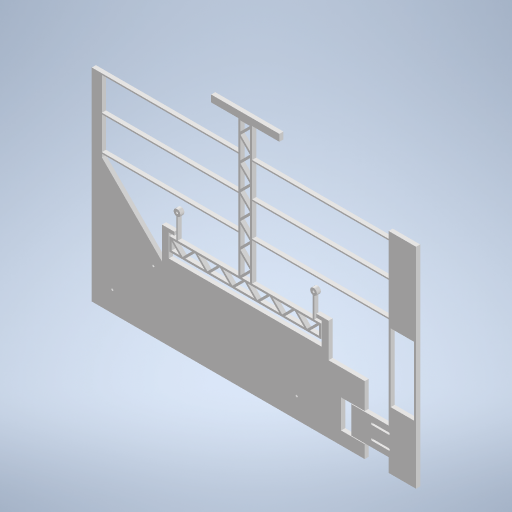
# Autodesk Inventor part: Inverter
Saved by Autodesk Inventor 2023 (Build 270158000, 158)
## iProperties
Created: 2023-05-11
Part Number: Inverter
Material: Generic
Document SubType Name: Modeling
Designer: Nathann
Density: 1 g/cm^3
Appearance: Default
Author: Nathann
Autodesk Inventor part; units mm, degrees
ref_plane "YZ Plane" through (0, 0, 0) normal (1, 0, 0) x (0, 1, 0)
ref_plane "XZ Plane" through (0, 0, 0) normal (0, 1, 0) x (-1, 0, 0)
ref_plane "XY Plane" through (0, 0, 0) normal (0, 0, 1) x (1, 0, 0)
sketch "Sketch1" plane through (0, 0, 0) normal (0, 0, 1) x (1, 0, 0)
  line L0 (0, 0) -> (-420, 0)
  line L1 (-420, 0) -> (-420, 350)
  line L2 (-420, 350) -> (0, 350)
  line L3 (0, 350) -> (0, 98.9027)
  line L4 (-98.9528, 98.9027) -> (-175.0251, 174.9749)
  line L5 (-175.0251, 174.9749) -> (0, 350)
  line L6 (-75.0251, 174.899) -> (-275.025, 174.899)
  circle A0 centre (-275.025, 174.899) radius 1.5
  circle A1 centre (-275.025, 174.899) radius 5
  circle A2 centre (-75.0251, 174.899) radius 5
  circle A3 centre (-75.0251, 174.899) radius 1.5
  line L7 (-274.025, 170) -> (-276.025, 170)
  line L8 (-276.025, 170) -> (-276.025, 140)
  line L9 (-276.025, 140) -> (-274.025, 140)
  line L10 (-274.025, 140) -> (-274.025, 170)
  line L11 (-74.0251, 170) -> (-76.0251, 170)
  line L12 (-76.0251, 170) -> (-76.0251, 140)
  line L13 (-76.0251, 140) -> (-74.0251, 140)
  line L14 (-74.0251, 140) -> (-74.0251, 170)
  line L15 (-64.0251, 140) -> (-286.025, 140)
  line L16 (-286.025, 140) -> (-286.025, 120)
  line L17 (-286.025, 120) -> (-64.0251, 120)
  line L18 (-64.0251, 120) -> (-64.0251, 140)
  line L19 (-165.0251, 140) -> (-185.0251, 140)
  line L20 (-185.0251, 140) -> (-185.0251, 340)
  line L21 (-185.0251, 340) -> (-165.0251, 340)
  line L22 (-165.0251, 340) -> (-165.0251, 140)
  line L23 (-185, 339) -> (-185.0251, 340)
  line L24 (-185.0251, 194.899) -> (-385.0251, 194.899)
  line L25 (-385.0251, 194.899) -> (-385.0251, 196.899)
  line L26 (-385.0251, 196.899) -> (-185.0251, 196.899)
  line L27 (-185.0251, 196.899) -> (-185.0251, 194.899)
  line L28 (-185.0251, 296.899) -> (-385.0251, 296.899)
  line L29 (-385.0251, 296.899) -> (-385.0251, 294.899)
  line L30 (-385.0251, 294.899) -> (-185.0251, 294.899)
  line L31 (-185.0251, 294.899) -> (-185.0251, 296.899)
  line L32 (-225.0251, 350) -> (-125.0251, 350)
  line L33 (-125.0251, 350) -> (-125.0251, 340)
  line L34 (-125.0251, 340) -> (-225.0251, 340)
  line L35 (-225.0251, 340) -> (-225.0251, 350)
  line L36 (-165.0251, 294.899) -> (34.9749, 294.899)
  line L37 (34.9749, 294.899) -> (34.9749, 296.899)
  line L38 (34.9749, 296.899) -> (-165.0251, 296.899)
  line L39 (-165.0251, 296.899) -> (-165.0251, 294.899)
  line L40 (0, 0) -> (135.1933, 0)
  line L41 (135.1933, 0) -> (135.1933, 350)
  line L42 (135.1933, 350) -> (0, 350)
  line L43 (0, 350) -> (0, 98.9027)
  line L44 (-165.0251, 196.899) -> (34.9749, 196.899)
  line L45 (34.9749, 196.899) -> (34.9749, 194.899)
  line L46 (34.9749, 194.899) -> (-165.0251, 194.899)
  line L47 (-165.0251, 194.899) -> (-165.0251, 196.899)
  line L48 (-420, 350) -> (-385, 350)
  line L49 (-385, 350) -> (-385, 98.9027)
  line L50 (-385, 98.9027) -> (-420, 98.9027)
  line L51 (-420, 98.9027) -> (-420, 350)
  line L52 (135.1933, 98.9027) -> (135.1933, 0)
  line L53 (135.1933, 0) -> (-420, 0)
  line L54 (-420, 0) -> (-420, 98.9027)
  line L55 (-185.0251, 246.899) -> (-385, 246.899)
  line L56 (-385, 246.899) -> (-385, 244.899)
  line L57 (-385, 244.899) -> (-185.0251, 244.899)
  line L58 (-185.0251, 244.899) -> (-185.0251, 246.899)
  line L59 (-165.0251, 246.899) -> (35, 246.899)
  line L60 (35, 246.899) -> (35, 244.899)
  line L61 (35, 244.899) -> (-165.0251, 244.899)
  line L62 (-165.0251, 244.899) -> (-165.0251, 246.899)
  line L63 (35, 306.899) -> (75, 306.899)
  line L64 (75, 306.899) -> (75, 184.899)
  line L65 (75, 184.899) -> (35, 184.899)
  line L66 (35, 184.899) -> (35, 306.899)
  line L67 (35, 184.899) -> (38, 184.899)
  line L68 (38, 184.899) -> (38, 84.899)
  line L69 (38, 84.899) -> (35, 84.899)
  line L70 (35, 84.899) -> (35, 184.899)
  line L71 (75, 184.899) -> (72, 184.899)
  line L72 (72, 184.899) -> (72, 84.899)
  line L73 (72, 84.899) -> (75, 84.899)
  line L74 (75, 84.899) -> (75, 184.899)
  line L75 (75, 84.899) -> (35, 84.899)
  line L76 (35, 84.899) -> (35, 0)
  line L77 (35, 0) -> (75, 0)
  line L78 (75, 0) -> (75, 84.899)
  line L79 (-420, 98.9027) -> (0, 98.9027)
  line L80 (35, 60) -> (-19.6162, 60)
  line L81 (-19.6162, 60) -> (-19.6162, 20)
  line L82 (-19.6162, 20) -> (35, 20)
  line L83 (35, 20) -> (35, 60)
  line L84 (0, 98.9027) -> (-37.8422, 98.9027)
  line L85 (-37.8422, 98.9027) -> (-37.8422, 61)
  line L86 (-37.8422, 61) -> (0, 61)
  line L87 (0, 61) -> (0, 98.9027)
  line L88 (-37.8422, 61) -> (-34.6162, 61)
  line L89 (-34.6162, 61) -> (-34.6162, 0)
  line L90 (-34.6162, 0) -> (-37.8422, 0)
  line L91 (-37.8422, 0) -> (-37.8422, 61)
  line L92 (-34.6162, 0) -> (0, 0)
  line L93 (0, 0) -> (0, 19)
  line L94 (0, 19) -> (-34.6162, 19)
  line L95 (-34.6162, 19) -> (-34.6162, 0)
  line L96 (-286.025, 98.9027) -> (-64.0251, 98.9027)
  line L97 (-64.0251, 98.9027) -> (-64.0251, 111)
  line L98 (-64.0251, 111) -> (-286.025, 111)
  line L99 (-286.025, 111) -> (-286.025, 98.9027)
  line L100 (-63.0251, 98.9027) -> (-53.0251, 98.9027)
  line L101 (-53.0251, 98.9027) -> (-53.0251, 140)
  line L102 (-53.0251, 140) -> (-63.0251, 140)
  line L103 (-63.0251, 140) -> (-63.0251, 98.9027)
  line L104 (-287.025, 98.9027) -> (-297.025, 98.9027)
  line L105 (-297.025, 98.9027) -> (-297.025, 140)
  line L106 (-297.025, 140) -> (-287.025, 140)
  line L107 (-287.025, 140) -> (-287.025, 98.9027)
  line L108 (-286.025, 111) -> (-287.025, 111)
  line L109 (-287.025, 111) -> (-287.025, 98.9027)
  line L110 (-287.025, 98.9027) -> (-286.025, 98.9027)
  line L111 (-286.025, 98.9027) -> (-286.025, 111)
  line L112 (-64.0251, 98.9027) -> (-63.0251, 98.9027)
  line L113 (-63.0251, 98.9027) -> (-63.0251, 111)
  line L114 (-63.0251, 111) -> (-64.0251, 111)
  line L115 (-64.0251, 111) -> (-64.0251, 98.9027)
  line L116 (-297.025, 140) -> (-287.025, 140)
  line L117 (-287.025, 140) -> (-287.025, 149)
  line L118 (-287.025, 149) -> (-297.025, 149)
  line L119 (-297.025, 149) -> (-297.025, 140)
  line L120 (-287.025, 149) -> (-279.025, 149)
  line L121 (-279.025, 149) -> (-279.025, 144)
  line L122 (-279.025, 144) -> (-287.025, 144)
  line L123 (-287.025, 144) -> (-287.025, 149)
  line L124 (-53.0251, 140) -> (-63.0251, 140)
  line L125 (-63.0251, 140) -> (-63.0251, 149)
  line L126 (-63.0251, 149) -> (-53.0251, 149)
  line L127 (-53.0251, 149) -> (-53.0251, 140)
  line L128 (-63.0251, 149) -> (-71.0251, 149)
  line L129 (-71.0251, 149) -> (-71.0251, 144)
  line L130 (-71.0251, 144) -> (-63.0251, 144)
  line L131 (-63.0251, 144) -> (-63.0251, 149)
  point P0 (-275.025, 140)
  point P1 (-175.0251, 174.899)
  point P2 (-175.0251, 340)
  point P3 (67.5967, 0)
  point P4 (-125.0251, 350)
  point P5 (-385, 296.899)
  point P6 (-385, 194.899)
  point P7 (-74.0251, 140)
  point P8 (-76.0251, 140)
  point P9 (35, 194.9749)
  point P10 (35, 296.9749)
  point P11 (35, 294.9749)
  point P12 (35, 246.899)
  point P13 (-185.0251, 294.899)
  point P14 (-385, 246.899)
  point P15 (-385, 294.899)
  point P16 (35, 244.899)
  point P17 (35, 196.9749)
  point P18 (38, 84.899)
  point P19 (38, 184.899)
  point P20 (72, 184.899)
  point P21 (72, 84.899)
  point P22 (-385, 196.899)
  point P23 (-185.0251, 244.899)
  point P24 (0, 194.899)
  point P25 (35, 84.899)
  point P26 (0, 350)
  point P27 (0, 296.899)
  point P28 (0, 196.899)
  point P29 (0, 294.899)
  point P30 (-64.0251, 98.9027)
  point P31 (-297.025, 98.9027)
  dimension "d9" = 10
  dimension "d0" = 420
  dimension "d1" = 350
  dimension "d2" = 45
  dimension "d3" = 45
  dimension "d4" = 100
  dimension "d5" = 100
  dimension "d6" = 3
  dimension "d7" = 3
  dimension "d8" = 10
  dimension "d10" = 1
  dimension "d11" = 2
  dimension "d12" = 30
  dimension "d13" = 30
  dimension "d14" = 2
  dimension "d15" = 20
  dimension "d16" = 10
  dimension "d23" = 10
  dimension "d24" = 10
  dimension "d25" = 10
  dimension "d26" = 200
  dimension "d28" = 2
  dimension "d29" = 200
  dimension "d30" = 2
  dimension "d31" = 200
  dimension "d32" = 100
  dimension "d33" = 20
  dimension "d34" = 10
  dimension "d35" = 40
  dimension "d36" = 40
  dimension "d37" = 200
  dimension "d38" = 200
  dimension "d39" = 2
  dimension "d40" = 2
  dimension "d41" = 100
  dimension "d42" = 2
  dimension "d43" = 50
  dimension "d44" = 40
  dimension "d45" = 10
  dimension "d46" = 10
  dimension "d47" = 50
  dimension "d48" = 100
  dimension "d49" = 3
  dimension "d50" = 3
  dimension "d54" = 1
  dimension "d55" = 1
  dimension "d56" = 40
  dimension "d57" = 15
  dimension "d58" = 20
  dimension "d66" = 9
  dimension "d69" = 2
  dimension "d121" = 0
  dimension "d122" = 0
  dimension "d123" = 10
  dimension "d124" = 10
  dimension "d125" = 1
  dimension "d126" = 1
  dimension "d127" = 5
  dimension "d128" = 4
  dimension "d129" = 5
  dimension "d130" = 3
  dimension "d131" = 3
  dimension "d132" = 4
  constraints: 264 end point, 63 parallel, 33 horizontal, 32 perpendicular, 22 point on line, 5 midpoint, 4 coincident, 3 centre point, 2 point on circle, 1 vertical, 3 other
  measures "d0" distance of L1.end L2.end
  measures "d1" distance of L2.end L0.start
  measures "d2" angle of L3 L5
  measures "d3" angle of L3 L4
  measures "d4" distance of L6.end L4.end
  measures "d5" distance of L6.start L4.end
  measures "d6" diameter of A3
  measures "d7" diameter of A0
  measures "d8" diameter of A2
  measures "d10" distance from line of L6.end L8
  measures "d11" distance between parallel lines of L10 L8
  measures "d12" distance of L7.end L8.end
  measures "d13" distance of L11.end L12.end
  measures "d14" distance between parallel lines of L14 L12
  measures "d15" distance between parallel lines of L17 L15
  measures "d16" distance between parallel lines of L8 L16
  measures "d23" distance between parallel lines of L18 L14
  measures "d24" distance from line of L22 point (-175.025, 174.899)
  measures "d25" distance from line of L20 L4.end
  measures "d26" distance between parallel lines of L15 L21
  measures "d28" distance between parallel lines of L24 L26
  measures "d29" distance of L25.end L26.end
  measures "d30" distance between parallel lines of L30 L28
  measures "d31" distance of L28.start L28.end
  measures "d32" distance between parallel lines of L28 L26
  measures "d33" distance from line of point (-275.025, 174.899) L24
  measures "d34" distance of L34.end L32.start
  measures "d35" distance between parallel lines of L20 L35
  measures "d36" distance between parallel lines of L33 L22
  measures "d37" distance of L36.start L36.end
  measures "d38" distance of L44.start L44.end
  measures "d39" distance between parallel lines of L44 L46
  measures "d40" distance between parallel lines of L36 L38
  measures "d41" distance between parallel lines of L46 L36
  measures "d42" distance between parallel lines of L57 L55
  measures "d43" distance between parallel lines of L55 L28
  measures "d44" distance of L63.start L63.end
  measures "d45" distance between parallel lines of L38 L63
  measures "d46" distance between parallel lines of L65 L46
  measures "d47" distance between parallel lines of L44 L59
  measures "d48" distance between parallel lines of L65 L69
  measures "d49" distance between parallel lines of L68 L70
  measures "d50" distance between parallel lines of L74 L72
  measures "d54" distance between parallel lines of L86 L80
  measures "d55" distance between parallel lines of L94 L82
  measures "d56" distance between parallel lines of L82 L80
  measures "d57" distance between parallel lines of L81 L89
  measures "d58" distance between parallel lines of L53 L82
  measures "d66" distance between parallel lines of L17 L98
  measures "d69" distance between parallel lines of L61 L59
  measures "d121" distance between parallel lines of L99 L16
  measures "d122" distance between parallel lines of L18 L97
  measures "d123" distance between parallel lines of L101 L103
  measures "d124" distance of L105.end L106.end
  measures "d125" distance between parallel lines of L16 L107
  measures "d126" distance between parallel lines of L103 L18
  measures "d127" distance of L120.end L121.end
  measures "d128" distance between parallel lines of L15 L122
  measures "d129" distance of L128.end L129.end
  measures "d130" distance between parallel lines of L14 L129
  measures "d131" distance between parallel lines of L8 L121
  measures "d132" distance between parallel lines of L15 L130
extrude "Extrusion1" add sketch "Sketch1" along normal blind 6 contours L0 L89 L94 L93 | L0 L91 L86 L89 | L76 L69 L75 L73 L78 L40 | L0 L1 L50 L79 L85 L91 | L82 L81 L80 L76 | L85 L79 L87 L86 | L73 L72 L65 L74 | L1 L2 L49 L28 L29 L30 L26 L25 L24 L50 | L65 L66 L60 L63 L64 | L70 L65 L68 L69 | L79 L103 L102 L101 | L49 L26 L20 L24 | L24 L25 L26 L49 | L105 L106 L107 L79 | L79 L97 L114 L103 | L102 L125 L126 L127 | L46 L5 L44 L3 | L3 L44 L45 L46 | L61 L3 L59 L60 | L2 L33 L34 L21 L35 | L49 L30 L29 L28 | L28 L20 L30 L49 | L20 L21 L22 L5 L4 L6 | L107 L108 L99 L79 | L119 L118 L117 L106 | L79 L4 L98 L97 | L46 L22 L44 L5 | L38 L37 L36 L3 | L3 L36 L5 L38 | L5 L36 L22 L38 | L61 L5 L59 L3 | L6 L4 L22 L15 L20 | L49 L55 L20 L57 | L99 L98 L4 L79 | L130 L129 L128 L125 | L22 L6 L4 L5 | L61 L22 L59 L5 | L6 L22 L4 | A1 L7 | L15 L4 L17 L16 L9 | L117 L120 L121 L122 | L7 A1 | A1 L10 L9 L8 | L4 L15 L13 L18 L17 | A2 L11 | L11 A2 | A2 L14 L13 L12
sketch "Sketch2" plane through (0, 0, 6) normal (0, 0, 1) x (1, 0, 0)
  line L0 (-399.7744, 175.1569) -> (-399.7744, 350.1556) projected
  line L1 (-420, 350) -> (-420, 0) projected
  line L2 (-399.7744, 350.1556) -> (-420, 350.1556)
  line L3 (-420, 350.1556) -> (-420, 0)
  line L4 (-420, 0) -> (-399.7744, 0)
  line L5 (-399.7744, 0) -> (-399.7744, 350.1556)
  line L6 (-385, 296.899) -> (-385, 350) projected
  line L7 (-399.7744, 350.1556) -> (-385, 350.1556)
  line L8 (-385, 350.1556) -> (-385, 296.899)
  line L9 (-385, 296.899) -> (-399.7744, 296.899)
  line L10 (-399.7744, 296.899) -> (-399.7744, 350.1556)
  point P0 (0, 0)
  point P1 (-399.7744, 296.899)
  constraints: 16 end point, 4 parallel, 2 horizontal, 2 perpendicular
extrude "Extrusion2" cut sketch "Sketch2" against normal blind 6
sketch "Sketch3" plane through (0, 0, 6) normal (0, 0, 1) x (1, 0, 0)
  line L0 (-385, 98.9027) -> (-385, 194.899) projected
  line L1 (-385, 190.2148) -> (-293.6879, 98.9027)
  line L2 (0, 98.9027) -> (-385, 98.9027) projected
  point P0 (0, 0)
  dimension "d61" = 45
  constraints: 2 end point, 2 point on line
  measures "d61" angle of L2 L1
extrude "Extrusion3" add sketch "Sketch3" against normal blind 6
sketch "Sketch4" plane through (0, 0, 6) normal (0, 0, 1) x (1, 0, 0)
  ellipse E0 centre (-99.7744, 30.1579) end of major axis (-101.2744, 30.1579) minor radius 1.5 projected
  ellipse E1 centre (-309.7744, 90.1575) end of major axis (-311.2744, 90.1575) minor radius 1.5 projected
  ellipse E2 centre (-369.7744, 30.1579) end of major axis (-371.2744, 30.1579) minor radius 1.5 projected
  line L0 (-239.7744, 310.1559) -> (-239.7744, 350.1556) projected
  line L1 (-307.6459, 350.1556) -> (-239.7744, 350.1556) projected
  line L2 (-307.6459, 341.1556) -> (-307.6459, 350.1556) projected
  line L3 (-274.7744, 341.1556) -> (-307.6459, 341.1556) projected
  line L4 (-274.7744, 309.1559) -> (-274.7744, 341.1556) projected
  line L5 (-307.6459, 309.1559) -> (-274.7744, 309.1559) projected
  line L6 (-307.6459, 195.1567) -> (-307.6459, 309.1559) projected
  line L7 (-297.6459, 195.1567) -> (-307.6459, 195.1567) projected
  line L8 (-297.6459, 185.1568) -> (-297.6459, 195.1567) projected
  line L9 (-285.3231, 185.1568) -> (-297.6459, 185.1568) projected
  ellipse E3 centre (-174.7744, 175.1569) end of major axis (-285.7744, 175.1569) minor radius 110.9992 (-103.6758, 260.397) -> (-285.3231, 185.1568) ccw projected
  line L10 (-26.5276, 337.5446) -> (-103.6758, 260.397) projected
  line L11 (-19.5768, 331.0605) -> (-26.5276, 337.5446) projected
  line L12 (-160.9903, 189.648) -> (-19.5768, 331.0605) projected
  ellipse E4 centre (-174.7744, 175.1569) end of major axis (-154.7744, 175.1569) minor radius 19.9999 (-160.9903, 189.648) -> (-169.598, 194.4752) ccw projected
  line L13 (-104.3858, 259.687) -> (-169.598, 194.4752) projected
  ellipse E5 centre (-174.7744, 175.1569) end of major axis (-64.7744, 175.1569) minor radius 109.9992 (-104.3858, 259.687) -> (-284.3189, 185.1568) ccw projected
  line L14 (-174.7744, 185.1568) -> (-284.3189, 185.1568) projected
  line L15 (-174.7744, 180.6568) -> (-174.7744, 185.1568) projected
  line L16 (-307.6459, 180.6568) -> (-174.7744, 180.6568) projected
  line L17 (-307.6459, 185.1568) -> (-307.6459, 180.6568) projected
  line L18 (-317.6459, 185.1568) -> (-307.6459, 185.1568) projected
  line L19 (-317.6459, 310.1559) -> (-317.6459, 185.1568) projected
  line L20 (-284.7744, 310.1559) -> (-317.6459, 310.1559) projected
  line L21 (-284.7744, 340.1556) -> (-284.7744, 310.1559) projected
  line L22 (-317.6459, 340.1556) -> (-284.7744, 340.1556) projected
  line L23 (-317.6459, 350.1556) -> (-317.6459, 340.1556) projected
  line L24 (-399.7744, 350.1556) -> (-317.6459, 350.1556) projected
  line L25 (-399.7744, 175.1569) -> (-399.7744, 350.1556) projected
  line L26 (-307.6459, 175.1569) -> (-399.7744, 175.1569) projected
  line L27 (-307.6459, 179.6568) -> (-307.6459, 175.1569) projected
  line L28 (-174.7744, 179.6568) -> (-307.6459, 179.6568) projected
  line L29 (-174.7744, 175.1569) -> (-174.7744, 179.6568) projected
  line L30 (-262.3486, 175.1569) -> (-174.7744, 175.1569) projected
  ellipse E6 centre (-274.8482, 175.0675) end of major axis (-287.3482, 175.0675) minor radius 12.4999 (-284.4789, 167.0988) -> (-262.3486, 175.1569) ccw projected
  ellipse E7 centre (-174.7744, 175.1569) end of major axis (-64.7744, 175.1569) minor radius 109.9992 (-284.4789, 167.0988) -> (-104.3858, 90.6268) ccw projected
  line L31 (-169.598, 155.8385) -> (-104.3858, 90.6268) projected
  ellipse E8 centre (-174.7744, 175.1569) end of major axis (-154.7744, 175.1569) minor radius 19.9999 (-169.598, 155.8385) -> (-160.9903, 160.6657) ccw projected
  line L32 (-19.5645, 19.241) -> (-160.9903, 160.6657) projected
  line L33 (-26.282, 12.5235) -> (-19.5645, 19.241) projected
  line L34 (-103.6758, 89.9167) -> (-26.282, 12.5235) projected
  ellipse E9 centre (-174.7744, 175.1569) end of major axis (-285.7744, 175.1569) minor radius 110.9992 (-285.5845, 168.6657) -> (-103.6758, 89.9167) ccw projected
  ellipse E10 centre (-274.8482, 175.0675) end of major axis (-287.3482, 175.0675) minor radius 12.4999 (-286.4769, 170.4823) -> (-285.5845, 168.6657) ccw projected
  line L35 (-399.7744, 170.4823) -> (-286.4769, 170.4823) projected
  line L36 (-399.7744, 0.1582) -> (-399.7744, 170.4823) projected
  line L37 (0.2256, 0.1582) -> (-399.7744, 0.1582) projected
  line L38 (0.2256, 350.1556) -> (0.2256, 0.1582) projected
  line L39 (-119.7744, 350.1556) -> (0.2256, 350.1556) projected
  line L40 (-119.7744, 350.1556) -> (-119.7744, 310.1559) projected
  line L41 (-119.7744, 310.1559) -> (-239.7744, 310.1559) projected
  line L42 (-160.2832, 161.3728) -> (-18.8574, 19.9481) projected
  ellipse E11 centre (-174.7744, 175.1569) end of major axis (-154.7744, 175.1569) minor radius 19.9999 (-160.2832, 161.3728) -> (-155.4559, 169.9805) ccw projected
  line L43 (-90.2437, 104.7688) -> (-155.4559, 169.9805) projected
  ellipse E12 centre (-174.7744, 175.1569) end of major axis (-64.7744, 175.1569) minor radius 109.9992 (-90.2437, 104.7688) -> (-90.2437, 245.5449) ccw projected
  line L44 (-155.4559, 180.3332) -> (-90.2437, 245.5449) projected
  ellipse E13 centre (-174.7744, 175.1569) end of major axis (-154.7744, 175.1569) minor radius 19.9999 (-155.4559, 180.3332) -> (-160.2832, 188.9409) ccw projected
  line L45 (-18.8451, 330.3779) -> (-160.2832, 188.9409) projected
  line L46 (-11.8942, 323.8938) -> (-18.8451, 330.3779) projected
  line L47 (-89.5337, 246.2549) -> (-11.8942, 323.8938) projected
  ellipse E14 centre (-174.7744, 175.1569) end of major axis (-285.7744, 175.1569) minor radius 110.9992 (-89.5337, 104.0588) -> (-89.5337, 246.2549) ccw projected
  line L48 (-12.1399, 26.6656) -> (-89.5337, 104.0588) projected
  line L49 (-18.8574, 19.9481) -> (-12.1399, 26.6656) projected
  line L50 (-397.5244, 195.1567) -> (-319.8959, 195.1567) projected
  line L51 (-397.5244, 295.156) -> (-397.5244, 195.1567) projected
  line L52 (-319.8959, 295.156) -> (-397.5244, 295.156) projected
  line L53 (-319.8959, 195.1567) -> (-319.8959, 295.156) projected
  ellipse E15 centre (-74.7744, 175.1569) end of major axis (-76.2744, 175.1569) minor radius 1.5 projected
  point P0 (0, 0)
  constraints: 16 other
extrude "Extrusion4" cut sketch "Sketch4" against normal blind 6 contours E0 | E1 | E2
sketch "Sketch6" plane through (0, 0, 6) normal (0, 0, 1) x (1, 0, 0)
  line L0 (35, 0) -> (75, 0) projected
  line L1 (75, 0) -> (75.2256, 0)
  line L2 (75.2256, 0) -> (75.2256, 306.9749)
  line L3 (75.2256, 306.9749) -> (75, 306.9749)
  line L4 (75, 306.9749) -> (75, 0)
  line L5 (-399.7744, 296.899) -> (-399.7744, 0) projected
  point P0 (0, 0)
  dimension "d70" = 475
  constraints: 8 end point, 2 parallel, 1 horizontal, 1 perpendicular
  measures "d70" distance between parallel lines of L5 L2
extrude "Extrusion6" add sketch "Sketch6" against normal blind 6
sketch "Sketch7" plane through (0, 0, 6) normal (0, 0, 1) x (1, 0, 0)
  circle A0 centre (35.2256, 30) radius 1.5
  circle A1 centre (35.2256, 50) radius 1.5
  line L0 (35, 0) -> (75.2256, 0) projected
  circle A2 centre (10.3838, 49.9999) radius 1.5
  circle A3 centre (10.3838, 30) radius 1.5
  line L1 (10.3991, 31.4999) -> (35.2256, 31.5)
  line L2 (35.3433, 28.5046) -> (10.5006, 28.5045)
  line L3 (10.3838, 48.4999) -> (35.2256, 48.5)
  line L4 (35.2256, 51.5) -> (10.3838, 51.4999)
  line L5 (75.2256, 0) -> (75.2256, 306.9749) projected
  line L6 (-19.6162, 60) -> (-19.6162, 20) projected
  point P0 (0, 0)
  dimension "d73" = 30
  dimension "d74" = 20
  dimension "d75" = 3
  dimension "d76" = 3
  dimension "d77" = 40
  dimension "d78" = 30
  dimension "d79" = 3
  dimension "d80" = 3
  dimension "d81" = 30
  dimension "d82" = 30
  constraints: 8 end point, 8 point on circle, 4 centre point, 3 parallel, 2 tangent, 1 vertical alignment
  measures "d73" distance from line of L0 A0.centre
  measures "d74" distance of A1.centre A0.centre
  measures "d75" diameter of A1
  measures "d76" diameter of A0
  measures "d77" distance from line of L5 A1.centre
  measures "d78" distance from line of L6 A2.centre
  measures "d79" diameter of A2
  measures "d80" diameter of A3
  measures "d81" distance from line of L6 A3.centre
  measures "d82" distance from line of A3.centre L0
extrude "Extrusion7" cut sketch "Sketch7" against normal blind 6
sketch "Sketch8" plane through (0, 0, 6) normal (0, 0, 1) x (1, 0, 0)
  line L0 (-283.025, 137) -> (-67.0251, 137)
  line L1 (-67.0251, 137) -> (-67.0251, 123)
  line L2 (-67.0251, 123) -> (-283.025, 123)
  line L3 (-283.025, 123) -> (-283.025, 137)
  line L4 (-185.0251, 140) -> (-274.025, 140) projected
  line L5 (-286.025, 120) -> (-64.0251, 120) projected
  line L6 (-286.025, 140) -> (-286.025, 120) projected
  line L7 (-64.0251, 120) -> (-64.0251, 140) projected
  line L8 (-283.025, 134.8787) -> (-271.1464, 123)
  line L9 (-280.9037, 137) -> (-266.9037, 123)
  line L10 (-266.9037, 123) -> (-252.9037, 137)
  line L11 (-262.6611, 123) -> (-248.6611, 137)
  line L12 (-248.6611, 137) -> (-234.6611, 123)
  line L13 (-230.4184, 123) -> (-244.4184, 137)
  line L14 (-230.4184, 123) -> (-216.4184, 137)
  line L15 (-226.1758, 123) -> (-212.1758, 137)
  line L16 (-193.9332, 123) -> (-207.9332, 137)
  line L17 (-212.1758, 137) -> (-198.1758, 123)
  line L18 (-193.9332, 123) -> (-179.9332, 137)
  line L19 (-189.6905, 123) -> (-175.6905, 137)
  line L20 (-157.4479, 123) -> (-171.4479, 137)
  line L21 (-175.6905, 137) -> (-161.6905, 123)
  line L22 (-157.4479, 123) -> (-143.4479, 137)
  line L23 (-153.2052, 123) -> (-139.2052, 137)
  line L24 (-120.9626, 123) -> (-134.9626, 137)
  line L25 (-139.2052, 137) -> (-125.2052, 123)
  line L26 (-120.9626, 123) -> (-106.9626, 137)
  line L27 (-116.7199, 123) -> (-102.7199, 137)
  line L28 (-84.4773, 123) -> (-98.4773, 137)
  line L29 (-102.7199, 137) -> (-88.7199, 123)
  line L30 (-84.4773, 123) -> (-70.4773, 137)
  line L31 (-80.2347, 123) -> (-66.2347, 137)
  line L32 (-47.992, 123) -> (-61.992, 137)
  line L33 (-66.2347, 137) -> (-52.2347, 123)
  line L34 (-67.0251, 136.2096) -> (-67.0251, 123)
  line L35 (-67.0251, 123) -> (-80.2347, 123)
  line L36 (-182.0251, 347) -> (-168.0251, 347)
  line L37 (-168.0251, 347) -> (-168.0251, 140)
  line L38 (-168.0251, 140) -> (-182.0251, 140)
  line L39 (-182.0251, 140) -> (-182.0251, 347)
  line L40 (-165.0251, 140) -> (-165.0251, 194.899) projected
  line L41 (-185.0251, 194.899) -> (-185.0251, 140) projected
  line L42 (-125.0251, 350) -> (-225.0251, 350) projected
  line L43 (-182.0251, 142.1213) -> (-168.0251, 156.1213)
  line L44 (-179.9037, 140) -> (-168.0251, 151.8787)
  line L45 (-168.0251, 156.1213) -> (-182.0251, 170.1213)
  line L46 (-182.0251, 174.364) -> (-168.0251, 160.364)
  line L47 (-182.0251, 174.364) -> (-168.0251, 188.364)
  line L48 (-182.0251, 178.6066) -> (-168.0251, 192.6066)
  line L49 (-168.0251, 192.6066) -> (-182.0251, 206.6066)
  line L50 (-182.0251, 210.8492) -> (-168.0251, 196.8492)
  line L51 (-182.0251, 210.8492) -> (-168.0251, 224.8492)
  line L52 (-182.0251, 215.0919) -> (-168.0251, 229.0919)
  line L53 (-168.0251, 229.0919) -> (-182.0251, 243.0919)
  line L54 (-182.0251, 247.3345) -> (-168.0251, 233.3345)
  line L55 (-182.0251, 247.3345) -> (-168.0251, 261.3345)
  line L56 (-182.0251, 251.5772) -> (-168.0251, 265.5772)
  line L57 (-168.0251, 265.5772) -> (-182.0251, 279.5772)
  line L58 (-182.0251, 283.8198) -> (-168.0251, 269.8198)
  line L59 (-182.0251, 283.8198) -> (-168.0251, 297.8198)
  line L60 (-182.0251, 288.0624) -> (-168.0251, 302.0624)
  line L61 (-168.0251, 302.0624) -> (-182.0251, 316.0624)
  line L62 (-182.0251, 320.3051) -> (-168.0251, 306.3051)
  line L63 (-182.0251, 320.3051) -> (-168.0251, 334.3051)
  line L64 (-182.0251, 324.5477) -> (-168.0251, 338.5477)
  line L65 (-168.0251, 338.5477) -> (-182.0251, 338.5477)
  point P0 (0, 0)
  point P1 (-80.2347, 123)
  point P2 (-98.4773, 137)
  point P3 (-88.7199, 123)
  point P4 (-116.7199, 123)
  point P5 (-125.2052, 123)
  point P6 (-153.2052, 123)
  point P7 (-226.1758, 123)
  point P8 (-189.6905, 123)
  point P9 (-168.0251, 192.6066)
  point P10 (-168.0251, 229.0919)
  point P11 (-168.0251, 265.5772)
  point P12 (-182.0251, 251.5772)
  point P13 (-168.0251, 302.0624)
  point P14 (-182.0251, 316.0624)
  point P15 (-182.0251, 338.5477)
  point P16 (-182.0251, 324.5477)
  dimension "d100" = 10
  dimension "d85" = 3
  dimension "d86" = 3
  dimension "d87" = 3
  dimension "d88" = 3
  dimension "d89" = 3
  dimension "d90" = 1.5
  dimension "d91" = 45
  dimension "d92" = 3
  dimension "d93" = 3
  dimension "d94" = 36.4853
  dimension "d97" = 36.4853
  dimension "d102" = 3
  dimension "d103" = 3
  dimension "d104" = 3
  dimension "d105" = 3
  dimension "d106" = 3
  dimension "d107" = 1.5
  dimension "d108" = 45
  dimension "d109" = 3
  dimension "d110" = 3
  dimension "d111" = 36.4853
  dimension "d114" = 36.4853
  constraints: 118 end point, 22 point on line, 10 parallel, 7 perpendicular, 4 horizontal, 1 collinear, 1 vertical, 99 other
  measures "d85" distance between parallel lines of L4 L0
  measures "d86" distance between parallel lines of L5 L2
  measures "d87" distance between parallel lines of L6 L3
  measures "d88" distance between parallel lines of L7 L1
  measures "d89" distance between parallel lines of L9 L8
  measures "d90" distance from line of L0.start L9
  measures "d91" angle of L0 L9
  measures "d92" distance between parallel lines of L11 L10
  measures "d93" distance between parallel lines of L12 L13
  measures "d94" distance of L13.start L9.end
  measures "d97" distance of L10.end L14.end
  measures "d102" distance between parallel lines of L40 L37
  measures "d103" distance between parallel lines of L41 L39
  measures "d104" distance between parallel lines of L0 L38
  measures "d105" distance between parallel lines of L42 L36
  measures "d106" distance between parallel lines of L43 L44
  measures "d107" distance from line of L44 L38.end
  measures "d108" angle of L38 L44
  measures "d109" distance between parallel lines of L46 L45
  measures "d110" distance between parallel lines of L47 L48
  measures "d111" distance of L43.end L48.end
  measures "d114" distance of L43.end L49.start
extrude "Extrusion8" cut sketch "Sketch8" against normal blind 10 contours L0 L10 L9 | L8 L2 L3 | L12 L2 L11 | L0 L14 L13 | L17 L2 L15 | L0 L18 L16 | L21 L2 L19 | L0 L22 L20 | L25 L2 L23 | L0 L26 L24 | L29 L2 L27 | L0 L30 L28 | L31 L1 L2 | L65 L64 L39 | L37 L62 L63 | L61 L60 L39 | L37 L58 L59 | L57 L56 L39 | L37 L54 L55 | L53 L52 L39 | L37 L50 L51 | L49 L48 L39 | L37 L46 L47 | L45 L43 L39 | L37 L38 L44
sketch "Sketch5" plane through (0, 0, 6) normal (0, 0, 1) x (1, 0, 0)
  line L0 (-385, 194.899) -> (-185.0251, 194.899) projected
  line L1 (-385, 196.899) -> (-385, 244.899) projected
  line L2 (-385, 194.899) -> (-385, 196.899)
  line L3 (-385, 244.899) -> (-185.0251, 244.899) projected
  line L4 (-385, 244.899) -> (-385, 246.899)
  line L5 (-385, 246.899) -> (-385, 294.899) projected
  line L6 (-385, 294.899) -> (-385, 296.899)
  line L7 (-185.0251, 296.899) -> (-399.7744, 296.899) projected
  line L8 (-165.0251, 194.899) -> (34.9749, 194.899) projected
  line L9 (34.9749, 196.899) -> (-165.0251, 196.899) projected
  line L10 (34.9749, 194.899) -> (34.9749, 196.899)
  line L11 (35, 244.899) -> (35, 196.899) projected
  line L12 (35, 246.899) -> (-165.0251, 246.899) projected
  line L13 (35, 244.899) -> (35, 246.899)
  line L14 (-165.0251, 294.899) -> (34.9749, 294.899) projected
  line L15 (34.9749, 294.899) -> (34.9749, 296.899)
  ellipse E0 centre (-99.7744, 30.1579) end of major axis (-101.2744, 30.1579) minor radius 1.5 projected
  ellipse E1 centre (-369.7744, 30.1579) end of major axis (-371.2744, 30.1579) minor radius 1.5 projected
  ellipse E2 centre (-309.7744, 90.1575) end of major axis (-311.2744, 90.1575) minor radius 1.5 projected
  line L16 (-399.7744, 295.9749) -> (-399.7744, 0) projected
  line L17 (-399.7744, 0) -> (0, 0) projected
  line L18 (0, 0) -> (0, 19) projected
  line L19 (0, 19) -> (-34.6162, 19) projected
  line L20 (-34.6162, 19) -> (-34.6162, 61) projected
  line L21 (-34.6162, 61) -> (0, 61) projected
  line L22 (0, 61) -> (0, 98.9027) projected
  line L23 (0, 98.9027) -> (-64.5, 98.9027) projected
  line L24 (-64.5, 98.9027) -> (-64.5, 111) projected
  line L25 (-64.5, 111) -> (-285, 111) projected
  line L26 (-285, 111) -> (-285, 98.9027) projected
  line L27 (-285, 98.9027) -> (-293.6879, 98.9027) projected
  line L28 (-293.6879, 98.9027) -> (-385, 190.2148) projected
  line L29 (-385, 190.2148) -> (-385, 194.9749) projected
  line L30 (-385, 194.9749) -> (-185, 194.9749) projected
  line L31 (-185, 194.9749) -> (-185, 140) projected
  line L32 (-185, 140) -> (-274.5, 140) projected
  line L33 (-274.5, 140) -> (-274.5, 170) projected
  arc A0 (-274.5, 170) -> (-275.5, 170) centre (-275, 174.9749) ccw projected
  line L34 (-275.5, 170) -> (-275.5, 140) projected
  line L35 (-275.5, 140) -> (-285.5, 140) projected
  line L36 (-285.5, 140) -> (-285.5, 120) projected
  line L37 (-285.5, 120) -> (-64.5, 120) projected
  line L38 (-64.5, 120) -> (-64.5, 140) projected
  line L39 (-64.5, 140) -> (-74.5, 140) projected
  line L40 (-74.5, 140) -> (-74.5, 170) projected
  arc A1 (-74.5, 170) -> (-75.5, 170) centre (-75, 174.9749) ccw projected
  line L41 (-75.5, 170) -> (-75.5, 140) projected
  line L42 (-75.5, 140) -> (-165, 140) projected
  line L43 (-165, 140) -> (-165, 194.9749) projected
  line L44 (-165, 194.9749) -> (35, 194.9749) projected
  line L45 (35, 194.9749) -> (35, 60) projected
  line L46 (35, 60) -> (-22.6162, 60) projected
  line L47 (-22.6162, 60) -> (-22.6162, 20) projected
  line L48 (-22.6162, 20) -> (35, 20) projected
  line L49 (35, 20) -> (35, 0) projected
  line L50 (35, 0) -> (75, 0) projected
  line L51 (75, 0) -> (75, 305.9749) projected
  line L52 (75, 305.9749) -> (35, 305.9749) projected
  line L53 (35, 305.9749) -> (35, 295.9749) projected
  line L54 (35, 295.9749) -> (-165, 295.9749) projected
  line L55 (-165, 295.9749) -> (-165, 340) projected
  line L56 (-165, 340) -> (-125, 340) projected
  line L57 (-125, 340) -> (-125, 350) projected
  line L58 (-125, 350) -> (-225, 350) projected
  line L59 (-225, 350) -> (-225, 340) projected
  line L60 (-225, 340) -> (-185, 340) projected
  line L61 (-185, 340) -> (-185, 295.9749) projected
  line L62 (-185, 295.9749) -> (-399.7744, 295.9749) projected
  line L63 (35, 245.9749) -> (-165, 245.9749) projected
  line L64 (-165, 245.9749) -> (-165, 294.9749) projected
  line L65 (-165, 294.9749) -> (35, 294.9749) projected
  line L66 (35, 294.9749) -> (35, 245.9749) projected
  line L67 (37, 84.9749) -> (37, 184.9749) projected
  line L68 (37, 184.9749) -> (73, 184.9749) projected
  line L69 (73, 184.9749) -> (73, 84.9749) projected
  line L70 (73, 84.9749) -> (37, 84.9749) projected
  line L71 (-185, 195.9749) -> (-385, 195.9749) projected
  line L72 (-385, 195.9749) -> (-385, 244.9749) projected
  line L73 (-385, 244.9749) -> (-185, 244.9749) projected
  line L74 (-185, 244.9749) -> (-185, 195.9749) projected
  line L75 (-185, 294.9749) -> (-185, 245.9749) projected
  line L76 (-185, 245.9749) -> (-385, 245.9749) projected
  line L77 (-385, 245.9749) -> (-385, 294.9749) projected
  line L78 (-385, 294.9749) -> (-185, 294.9749) projected
  circle A2 centre (-75, 174.9749) radius 1.5 projected
  circle A3 centre (-275, 174.9749) radius 1.5 projected
  line L79 (35, 195.9749) -> (-165, 195.9749) projected
  line L80 (-165, 195.9749) -> (-165, 244.9749) projected
  line L81 (-165, 244.9749) -> (35, 244.9749) projected
  line L82 (35, 244.9749) -> (35, 195.9749) projected
  constraints: 12 end point, 4 vertical, 1 coincident, 1 collinear, 1 point on line, 3 other
equation "\"d5\" = d4"
equation "\"d7\" = d6"
equation "\"d16\" = d23"
equation "\"d25\" = d24"
equation "\"d50\" = d49"
equation "\"bladeThicknessTablePushing\" = 1"
equation "\"bladeThicknessTable\" = 1"
equation "\"bladeThicknessForceConverter\" = 2"
equation "\"bladeThicknessWheelAnchor\" = 1"
equation "\"BladeThicknessRCC\" = 1"
equation "\"bladeThicknessZeroConverter\" = 2.25"
equation "\"rangeXProbeMax\" = 1"
equation "\"rangeXProbeMin\" = -1"
equation "\"safetyPlay\" = 0.1"
equation "\"OffsetMotorSpring\" = -1"
equation "\"thicknessWheelPlate\" = 6"
equation "\"thicknessConverterPlate\" = 6"
body "Solid1"
